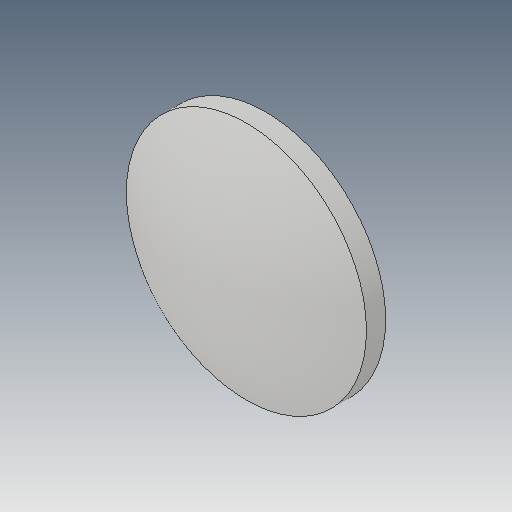
# Autodesk Inventor part: 30_CUBE_openSIM_Beamexpander_Lens_15mm
Saved by Autodesk Inventor 2019 (Build 230136000, 136)
## iProperties
Created: 2019-10-22
Part Number: 30_CUBE_openSIM_Beamexpander_Lens_15mm
Material: Generic
Document SubType Name: Modeling
Designer: diederichbenedict
Density: 1 g/cm^3
Appearance: Default
Author: diederichbenedict
Autodesk Inventor part; units mm, degrees
ref_plane "YZ Plane" through (0, 0, 0) normal (1, 0, 0) x (0, 1, 0)
ref_plane "XZ Plane" through (0, 0, 0) normal (0, 1, 0) x (-1, 0, 0)
ref_plane "XY Plane" through (0, 0, 0) normal (0, 0, 1) x (1, 0, 0)
sketch "Sketch1" plane through (0, 0, 0) normal (0, 1, 0) x (-1, 0, 0)
  line L0 (-7.331, -4.7098) -> (-7.331, -6.7098) projected
  line L1 (-7.331, -9.4466) -> (-7.331, -6.7098) projected
  spline S0 degree 3 poles (7.0432, -4.7098) (6.9856, -4.6712) (6.9277, -4.633) (6.2569, -4.1986) (5.6091, -3.8575) (4.9604, -3.5892) (4.9156, -3.571) (4.8706, -3.5532) knots 1.313478 1.313478 1.313478 1.313478 1.332863 1.332863 1.536826 1.536826 1.551818 1.551818 1.551818 1.551818 construction
  arc A0 (2.913, -9.4466) -> (8.1465, -6.7098) centre (-4.3535, 10.8214) ccw construction
  spline S1 degree 3 poles (7.0432, -4.7098) (6.9856, -4.6712) (6.9277, -4.633) (6.2569, -4.1986) (5.6091, -3.8575) (4.9604, -3.5892) (4.9156, -3.571) (4.8706, -3.5532) knots 1.313478 1.313478 1.313478 1.313478 1.332863 1.332863 1.536826 1.536826 1.551818 1.551818 1.551818 1.551818 construction
  arc A1 (8.1465, -4.7098) -> (6.3404, -3.5532) centre (-4.3535, -22.2411) ccw
  line L2 (8.1465, -6.7098) -> (-4.3535, -6.7098)
  line L3 (-4.3535, -6.7098) -> (-4.3535, -4.7098)
  line L4 (-4.3535, -4.7098) -> (8.1465, -4.7098)
  line L5 (8.1465, -4.7098) -> (8.1465, -6.7098)
  arc A2 (-4.3535, -10.7098) -> (8.1465, -6.7098) centre (-4.3535, 10.8214) ccw
  arc A3 (8.1465, -4.7098) -> (-4.3535, -0.7098) centre (-4.3535, -22.2411) ccw
  line L6 (-4.3535, -10.7098) -> (-4.3535, -6.7098)
  line L7 (-4.3535, -4.7098) -> (-4.3535, -0.7098)
  point P0 (0, 0)
  constraints: 12 end point, 9 point on circle, 4 centre point, 3 equal length, 2 concentric, 1 horizontal, 1 perpendicular, 1 vertical, 8 other
revolve "Revolution1" add sketch "Sketch1" angle 360 about axis through (4.3535, 0, -4.7098) along (0, 0, 1)
body "Solid1"
